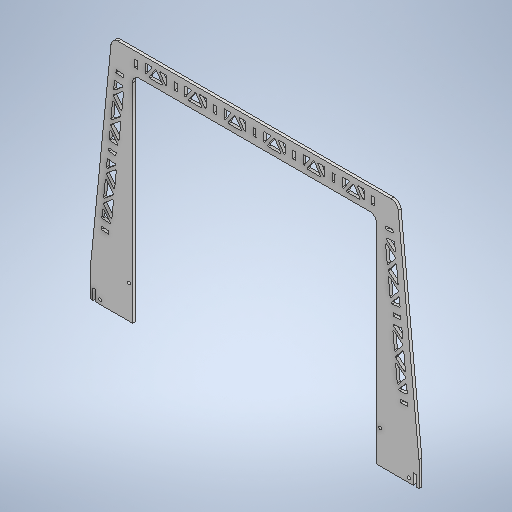
# Autodesk Inventor part: GateBrigeSide
Saved by Autodesk Inventor 2025.1 (Build 291241000, 241)
## iProperties
Created: 2025-03-30
Part Number: GateBrigeSide
Material: Všeobecné
Document SubType Name: Modeling
Designer: 42060
Density: 1 g/cm^3
Appearance: Výchozí
Author: 42060
Autodesk Inventor part; units mm, degrees
ref_plane "YZ Plane" through (0, 0, 0) normal (1, 0, 0) x (0, 1, 0)
ref_plane "XZ Plane" through (0, 0, 0) normal (0, 1, 0) x (-1, 0, 0)
ref_plane "XY Plane" through (0, 0, 0) normal (0, 0, 1) x (1, 0, 0)
sketch "Náčrt1" plane through (0, 0, 0) normal (0, 0, 1) x (1, 0, 0)
  line L0 (0, 0) -> (-160, 0)
  line L1 (-170, -10) -> (-170, -300)
  line L2 (-229, -300) -> (-229, -265.3)
  line L3 (-190.0509, 30) -> (0, 30)
  line L4 (0, 30) -> (0, 0)
  line L5 (-203.7, -249) -> (-170, -249)
  line L6 (-170, -249) -> (-170, -299)
  line L7 (-170, -299) -> (-220, -299)
  line L8 (-220, -299) -> (-220, -265.3)
  line L9 (-220, -265.3) -> (-203.7, -249)
  line L10 (-220, -299) -> (-170, -249) construction
  circle A0 centre (-215, -294) radius 2.1
  circle A1 centre (-175, -254) radius 2.1
  arc A2 (-160, 0) -> (-170, -10) centre (-160, -10) ccw
  line L11 (-200, 21.0077) -> (-229, -265.3)
  arc A3 (-190.0509, 30) -> (-200, 21.0077) centre (-190.0509, 20) ccw
  line L12 (-225, -300) -> (-225, -285)
  line L13 (-225, -285) -> (-221, -285)
  line L14 (-221, -285) -> (-221, -300)
  line L15 (-170, -300) -> (-221, -300)
  line L16 (-225, -300) -> (-229, -300)
  line L17 (-2, 10) -> (2, 10)
  line L18 (2, 10) -> (2, 20)
  line L19 (2, 20) -> (-2, 20)
  line L20 (-2, 20) -> (-2, 10)
  line L21 (-57, 20) -> (-57, 10)
  line L22 (-53, 20) -> (-57, 20)
  line L23 (-53, 10) -> (-53, 20)
  line L24 (-57, 10) -> (-53, 10)
  line L25 (-112, 20) -> (-112, 10)
  line L26 (-108, 20) -> (-112, 20)
  line L27 (-108, 10) -> (-108, 20)
  line L28 (-112, 10) -> (-108, 10)
  line L29 (-167, 20) -> (-167, 10)
  line L30 (-163, 20) -> (-167, 20)
  line L31 (-163, 10) -> (-163, 20)
  line L32 (-167, 10) -> (-163, 10)
  line L33 (-192.6355, -5.5165) -> (-182.6864, -6.5242)
  line L34 (-182.6864, -6.5242) -> (-183.0895, -10.5039)
  line L35 (-183.0895, -10.5039) -> (-193.0386, -9.4961)
  line L36 (-193.0386, -9.4961) -> (-192.6355, -5.5165)
  line L37 (-193.1669, -109.9948) -> (-203.116, -108.9871)
  line L38 (-192.7638, -106.0152) -> (-193.1669, -109.9948)
  line L39 (-203.116, -108.9871) -> (-202.7129, -105.0074)
  line L40 (-202.7129, -105.0074) -> (-192.7638, -106.0152)
  line L41 (-203.2443, -209.4857) -> (-213.1934, -208.478)
  line L42 (-202.8412, -205.5061) -> (-203.2443, -209.4857)
  line L43 (-213.1934, -208.478) -> (-212.7903, -204.4984)
  line L44 (-212.7903, -204.4984) -> (-202.8412, -205.5061)
  line L45 (0, 0) -> (160, 0)
  line L46 (170, -10) -> (170, -300)
  line L47 (229, -300) -> (229, -265.3)
  line L48 (190.0509, 30) -> (0, 30)
  line L49 (203.7, -249) -> (170, -249)
  line L50 (170, -249) -> (170, -299)
  line L51 (170, -299) -> (220, -299)
  line L52 (220, -299) -> (220, -265.3)
  line L53 (220, -265.3) -> (203.7, -249)
  line L54 (220, -299) -> (170, -249) construction
  circle A4 centre (215, -294) radius 2.1
  circle A5 centre (175, -254) radius 2.1
  arc A6 (170, -10) -> (160, 0) centre (160, -10) ccw
  line L55 (200, 21.0077) -> (229, -265.3)
  arc A7 (200, 21.0077) -> (190.0509, 30) centre (190.0509, 20) ccw
  line L56 (225, -300) -> (225, -285)
  line L57 (225, -285) -> (221, -285)
  line L58 (221, -285) -> (221, -300)
  line L59 (170, -300) -> (221, -300)
  line L60 (225, -300) -> (229, -300)
  line L61 (2, 10) -> (-2, 10)
  line L62 (-2, 10) -> (-2, 20)
  line L63 (-2, 20) -> (2, 20)
  line L64 (2, 20) -> (2, 10)
  line L65 (57, 20) -> (57, 10)
  line L66 (53, 20) -> (57, 20)
  line L67 (53, 10) -> (53, 20)
  line L68 (57, 10) -> (53, 10)
  line L69 (112, 20) -> (112, 10)
  line L70 (108, 20) -> (112, 20)
  line L71 (108, 10) -> (108, 20)
  line L72 (112, 10) -> (108, 10)
  line L73 (167, 20) -> (167, 10)
  line L74 (163, 20) -> (167, 20)
  line L75 (163, 10) -> (163, 20)
  line L76 (167, 10) -> (163, 10)
  line L77 (192.6355, -5.5165) -> (182.6864, -6.5242)
  line L78 (182.6864, -6.5242) -> (183.0895, -10.5039)
  line L79 (183.0895, -10.5039) -> (193.0386, -9.4961)
  line L80 (193.0386, -9.4961) -> (192.6355, -5.5165)
  line L81 (193.1669, -109.9948) -> (203.116, -108.9871)
  line L82 (192.7638, -106.0152) -> (193.1669, -109.9948)
  line L83 (203.116, -108.9871) -> (202.7129, -105.0074)
  line L84 (202.7129, -105.0074) -> (192.7638, -106.0152)
  line L85 (203.2443, -209.4857) -> (213.1934, -208.478)
  line L86 (202.8412, -205.5061) -> (203.2443, -209.4857)
  line L87 (213.1934, -208.478) -> (212.7903, -204.4984)
  line L88 (212.7903, -204.4984) -> (202.8412, -205.5061)
  line L89 (-36.6095, 9.0611) -> (-28.3278, 21.2788)
  line L90 (-26.6722, 21.2788) -> (-18.3905, 9.0611)
  line L91 (-19.2183, 7.5) -> (-35.7817, 7.5)
  line L92 (-21.6095, 20.9389) -> (-14.3278, 10.1964)
  line L93 (-12.5, 10.7575) -> (-12.5, 21.5)
  line L94 (-13.5, 22.5) -> (-20.7817, 22.5)
  line L95 (-33.3905, 20.9389) -> (-40.6722, 10.1964)
  line L96 (-42.5, 10.7575) -> (-42.5, 21.5)
  line L97 (-41.5, 22.5) -> (-34.2183, 22.5)
  line L98 (-53, 15) -> (-2, 15) construction
  arc A8 (-41.5, 22.5) -> (-42.5, 21.5) centre (-41.5, 21.5) ccw
  arc A9 (-33.3905, 20.9389) -> (-34.2183, 22.5) centre (-34.2183, 21.5) ccw
  arc A10 (-42.5, 10.7575) -> (-40.6722, 10.1964) centre (-41.5, 10.7575) ccw
  arc A11 (-36.6095, 9.0611) -> (-35.7817, 7.5) centre (-35.7817, 8.5) ccw
  arc A12 (-19.2183, 7.5) -> (-18.3905, 9.0611) centre (-19.2183, 8.5) ccw
  arc A13 (-26.6722, 21.2788) -> (-28.3278, 21.2788) centre (-27.5, 20.7178) ccw
  arc A14 (-20.7817, 22.5) -> (-21.6095, 20.9389) centre (-20.7817, 21.5) ccw
  arc A15 (-12.5, 21.5) -> (-13.5, 22.5) centre (-13.5, 21.5) ccw
  arc A16 (-14.3278, 10.1964) -> (-12.5, 10.7575) centre (-13.5, 10.7575) ccw
  arc A17 (-81.6722, 21.2788) -> (-83.3278, 21.2788) centre (-82.5, 20.7178) ccw
  line L99 (-91.6095, 9.0611) -> (-83.3278, 21.2788)
  line L100 (-68.5, 22.5) -> (-75.7817, 22.5)
  arc A18 (-67.5, 21.5) -> (-68.5, 22.5) centre (-68.5, 21.5) ccw
  line L101 (-81.6722, 21.2788) -> (-73.3905, 9.0611)
  arc A19 (-74.2183, 7.5) -> (-73.3905, 9.0611) centre (-74.2183, 8.5) ccw
  line L102 (-76.6095, 20.9389) -> (-69.3278, 10.1964)
  line L103 (-74.2183, 7.5) -> (-90.7817, 7.5)
  arc A20 (-69.3278, 10.1964) -> (-67.5, 10.7575) centre (-68.5, 10.7575) ccw
  line L104 (-108, 15) -> (-57, 15) construction
  arc A21 (-96.5, 22.5) -> (-97.5, 21.5) centre (-96.5, 21.5) ccw
  arc A22 (-97.5, 10.7575) -> (-95.6722, 10.1964) centre (-96.5, 10.7575) ccw
  arc A23 (-91.6095, 9.0611) -> (-90.7817, 7.5) centre (-90.7817, 8.5) ccw
  arc A24 (-88.3905, 20.9389) -> (-89.2183, 22.5) centre (-89.2183, 21.5) ccw
  line L105 (-67.5, 10.7575) -> (-67.5, 21.5)
  arc A25 (-75.7817, 22.5) -> (-76.6095, 20.9389) centre (-75.7817, 21.5) ccw
  line L106 (-96.5, 22.5) -> (-89.2183, 22.5)
  line L107 (-88.3905, 20.9389) -> (-95.6722, 10.1964)
  line L108 (-97.5, 10.7575) -> (-97.5, 21.5)
  arc A26 (-136.6722, 21.2788) -> (-138.3278, 21.2788) centre (-137.5, 20.7178) ccw
  line L109 (-146.6095, 9.0611) -> (-138.3278, 21.2788)
  line L110 (-123.5, 22.5) -> (-130.7817, 22.5)
  arc A27 (-122.5, 21.5) -> (-123.5, 22.5) centre (-123.5, 21.5) ccw
  line L111 (-136.6722, 21.2788) -> (-128.3905, 9.0611)
  arc A28 (-129.2183, 7.5) -> (-128.3905, 9.0611) centre (-129.2183, 8.5) ccw
  line L112 (-131.6095, 20.9389) -> (-124.3278, 10.1964)
  line L113 (-129.2183, 7.5) -> (-145.7817, 7.5)
  arc A29 (-124.3278, 10.1964) -> (-122.5, 10.7575) centre (-123.5, 10.7575) ccw
  line L114 (-163, 15) -> (-112, 15) construction
  arc A30 (-151.5, 22.5) -> (-152.5, 21.5) centre (-151.5, 21.5) ccw
  arc A31 (-152.5, 10.7575) -> (-150.6722, 10.1964) centre (-151.5, 10.7575) ccw
  arc A32 (-146.6095, 9.0611) -> (-145.7817, 7.5) centre (-145.7817, 8.5) ccw
  arc A33 (-143.3905, 20.9389) -> (-144.2183, 22.5) centre (-144.2183, 21.5) ccw
  line L115 (-122.5, 10.7575) -> (-122.5, 21.5)
  arc A34 (-130.7817, 22.5) -> (-131.6095, 20.9389) centre (-130.7817, 21.5) ccw
  line L116 (-151.5, 22.5) -> (-144.2183, 22.5)
  line L117 (-143.3905, 20.9389) -> (-150.6722, 10.1964)
  line L118 (-152.5, 10.7575) -> (-152.5, 21.5)
  line L119 (-194.0109, -19.4488) -> (-184.1326, -20.4494)
  line L120 (-183.6011, -22.2191) -> (-194.48, -31.0969)
  line L121 (-196.1072, -30.2213) -> (-195.1066, -20.3429)
  line L122 (-182.544, -28.7227) -> (-184.7467, -50.4692)
  line L123 (-186.5164, -51.0007) -> (-196.2883, -39.0261)
  line L124 (-196.1458, -37.6191) -> (-184.1711, -27.8471)
  line L125 (-195.9642, -45.7498) -> (-186.1923, -57.7245)
  line L126 (-186.3348, -59.1315) -> (-198.3095, -68.9034)
  line L127 (-199.9366, -68.0279) -> (-197.7339, -46.2813)
  line L128 (-188.0006, -65.6537) -> (-199.9752, -75.4256)
  line L129 (-200.1177, -76.8326) -> (-190.3458, -88.8073)
  line L130 (-188.5761, -88.2758) -> (-186.3734, -66.5292)
  line L131 (-199.7937, -83.5564) -> (-190.9158, -94.4353)
  line L132 (-191.7914, -96.0625) -> (-201.6698, -95.0619)
  line L133 (-202.5639, -93.9662) -> (-201.5633, -84.0878)
  line L134 (-189.0718, -19.9491) -> (-188.064, -10) construction
  arc A35 (-194.0109, -19.4488) -> (-195.1066, -20.3429) centre (-194.1117, -20.4437) ccw
  arc A36 (-183.6011, -22.2191) -> (-184.1326, -20.4494) centre (-184.2333, -21.4443) ccw
  arc A37 (-196.1072, -30.2213) -> (-194.48, -31.0969) centre (-195.1123, -30.3221) ccw
  arc A38 (-196.1458, -37.6191) -> (-196.2883, -39.0261) centre (-195.5135, -38.3938) ccw
  arc A39 (-186.5164, -51.0007) -> (-184.7467, -50.4692) centre (-185.7416, -50.3685) ccw
  arc A40 (-182.544, -28.7227) -> (-184.1711, -27.8471) centre (-183.5389, -28.6219) ccw
  arc A41 (-195.9642, -45.7498) -> (-197.7339, -46.2813) centre (-196.739, -46.3821) ccw
  arc A42 (-186.3348, -59.1315) -> (-186.1923, -57.7245) centre (-186.9671, -58.3567) ccw
  arc A43 (-199.9366, -68.0279) -> (-198.3095, -68.9034) centre (-198.9417, -68.1287) ccw
  arc A44 (-199.9752, -75.4256) -> (-200.1177, -76.8326) centre (-199.343, -76.2004) ccw
  arc A45 (-190.3458, -88.8073) -> (-188.5761, -88.2758) centre (-189.571, -88.175) ccw
  arc A46 (-186.3734, -66.5292) -> (-188.0006, -65.6537) centre (-187.3683, -66.4284) ccw
  arc A47 (-199.7937, -83.5564) -> (-201.5633, -84.0878) centre (-200.5684, -84.1886) ccw
  arc A48 (-202.5639, -93.9662) -> (-201.6698, -95.0619) centre (-201.569, -94.067) ccw
  arc A49 (-191.7914, -96.0625) -> (-190.9158, -94.4353) centre (-191.6906, -95.0676) ccw
  arc A50 (-212.6413, -193.4572) -> (-211.7472, -194.5528) centre (-211.6464, -193.5579) ccw
  line L135 (-201.8688, -195.5534) -> (-211.7472, -194.5528)
  arc A51 (-201.8688, -195.5534) -> (-200.9932, -193.9263) centre (-201.768, -194.5585) ccw
  arc A52 (-200.4232, -188.2982) -> (-198.6535, -187.7667) centre (-199.6484, -187.666) ccw
  line L136 (-209.871, -183.0473) -> (-200.9932, -193.9263)
  line L137 (-212.6413, -193.4572) -> (-211.6407, -183.5788)
  arc A53 (-209.871, -183.0473) -> (-211.6407, -183.5788) centre (-210.6458, -183.6796) ccw
  line L138 (-198.078, -165.1446) -> (-210.0526, -174.9165)
  line L139 (-210.1951, -176.3236) -> (-200.4232, -188.2982)
  line L140 (-198.6535, -187.7667) -> (-196.4508, -166.0201)
  arc A54 (-210.0526, -174.9165) -> (-210.1951, -176.3236) centre (-209.4204, -175.6913) ccw
  arc A55 (-210.014, -167.5188) -> (-208.3869, -168.3944) centre (-209.0191, -167.6196) ccw
  arc A56 (-196.4508, -166.0201) -> (-198.078, -165.1446) centre (-197.4457, -165.9194) ccw
  line L141 (-206.0416, -145.2407) -> (-196.2697, -157.2154)
  arc A57 (-196.4122, -158.6224) -> (-196.2697, -157.2154) centre (-197.0445, -157.8476) ccw
  line L142 (-210.014, -167.5188) -> (-207.8113, -145.7722)
  line L143 (-196.4122, -158.6224) -> (-208.3869, -168.3944)
  arc A58 (-196.5938, -150.4917) -> (-194.8241, -149.9602) centre (-195.819, -149.8594) ccw
  arc A59 (-206.0416, -145.2407) -> (-207.8113, -145.7722) centre (-206.8164, -145.873) ccw
  line L144 (-196.5938, -150.4917) -> (-206.3657, -138.517)
  arc A60 (-206.2232, -137.11) -> (-206.3657, -138.517) centre (-205.5909, -137.8848) ccw
  arc A61 (-206.1846, -129.7123) -> (-204.5574, -130.5878) centre (-205.1897, -129.813) ccw
  line L145 (-192.6214, -128.2136) -> (-194.8241, -149.9602)
  line L146 (-206.2232, -137.11) -> (-194.2485, -127.338)
  arc A62 (-192.6214, -128.2136) -> (-194.2485, -127.338) centre (-193.6163, -128.1128) ccw
  arc A63 (-193.6785, -121.71) -> (-194.21, -119.9403) centre (-194.3107, -120.9352) ccw
  line L147 (-199.1491, -119.44) -> (-198.1414, -109.4909) construction
  line L148 (-204.0883, -118.9397) -> (-194.21, -119.9403)
  arc A64 (-204.0883, -118.9397) -> (-205.184, -119.8339) centre (-204.1891, -119.9346) ccw
  line L149 (-193.6785, -121.71) -> (-204.5574, -130.5878)
  line L150 (-206.1846, -129.7123) -> (-205.184, -119.8339)
  line L151 (36.6095, 9.0611) -> (28.3278, 21.2788)
  line L152 (26.6722, 21.2788) -> (18.3905, 9.0611)
  line L153 (19.2183, 7.5) -> (35.7817, 7.5)
  line L154 (21.6095, 20.9389) -> (14.3278, 10.1964)
  line L155 (12.5, 10.7575) -> (12.5, 21.5)
  line L156 (13.5, 22.5) -> (20.7817, 22.5)
  line L157 (33.3905, 20.9389) -> (40.6722, 10.1964)
  line L158 (42.5, 10.7575) -> (42.5, 21.5)
  line L159 (41.5, 22.5) -> (34.2183, 22.5)
  line L160 (53, 15) -> (2, 15) construction
  arc A65 (42.5, 21.5) -> (41.5, 22.5) centre (41.5, 21.5) ccw
  arc A66 (34.2183, 22.5) -> (33.3905, 20.9389) centre (34.2183, 21.5) ccw
  arc A67 (40.6722, 10.1964) -> (42.5, 10.7575) centre (41.5, 10.7575) ccw
  arc A68 (35.7817, 7.5) -> (36.6095, 9.0611) centre (35.7817, 8.5) ccw
  arc A69 (18.3905, 9.0611) -> (19.2183, 7.5) centre (19.2183, 8.5) ccw
  arc A70 (28.3278, 21.2788) -> (26.6722, 21.2788) centre (27.5, 20.7178) ccw
  arc A71 (21.6095, 20.9389) -> (20.7817, 22.5) centre (20.7817, 21.5) ccw
  arc A72 (13.5, 22.5) -> (12.5, 21.5) centre (13.5, 21.5) ccw
  arc A73 (12.5, 10.7575) -> (14.3278, 10.1964) centre (13.5, 10.7575) ccw
  line L161 (67.5, 10.7575) -> (67.5, 21.5)
  line L162 (96.5, 22.5) -> (89.2183, 22.5)
  arc A74 (97.5, 21.5) -> (96.5, 22.5) centre (96.5, 21.5) ccw
  line L163 (97.5, 10.7575) -> (97.5, 21.5)
  arc A75 (95.6722, 10.1964) -> (97.5, 10.7575) centre (96.5, 10.7575) ccw
  arc A76 (67.5, 10.7575) -> (69.3278, 10.1964) centre (68.5, 10.7575) ccw
  arc A77 (68.5, 22.5) -> (67.5, 21.5) centre (68.5, 21.5) ccw
  arc A78 (89.2183, 22.5) -> (88.3905, 20.9389) centre (89.2183, 21.5) ccw
  arc A79 (83.3278, 21.2788) -> (81.6722, 21.2788) centre (82.5, 20.7178) ccw
  line L164 (88.3905, 20.9389) -> (95.6722, 10.1964)
  line L165 (91.6095, 9.0611) -> (83.3278, 21.2788)
  arc A80 (76.6095, 20.9389) -> (75.7817, 22.5) centre (75.7817, 21.5) ccw
  arc A81 (90.7817, 7.5) -> (91.6095, 9.0611) centre (90.7817, 8.5) ccw
  line L166 (108, 15) -> (57, 15) construction
  line L167 (68.5, 22.5) -> (75.7817, 22.5)
  line L168 (76.6095, 20.9389) -> (69.3278, 10.1964)
  line L169 (81.6722, 21.2788) -> (73.3905, 9.0611)
  arc A82 (73.3905, 9.0611) -> (74.2183, 7.5) centre (74.2183, 8.5) ccw
  line L170 (74.2183, 7.5) -> (90.7817, 7.5)
  line L171 (122.5, 10.7575) -> (122.5, 21.5)
  line L172 (151.5, 22.5) -> (144.2183, 22.5)
  arc A83 (152.5, 21.5) -> (151.5, 22.5) centre (151.5, 21.5) ccw
  line L173 (152.5, 10.7575) -> (152.5, 21.5)
  arc A84 (150.6722, 10.1964) -> (152.5, 10.7575) centre (151.5, 10.7575) ccw
  arc A85 (122.5, 10.7575) -> (124.3278, 10.1964) centre (123.5, 10.7575) ccw
  arc A86 (123.5, 22.5) -> (122.5, 21.5) centre (123.5, 21.5) ccw
  arc A87 (144.2183, 22.5) -> (143.3905, 20.9389) centre (144.2183, 21.5) ccw
  arc A88 (138.3278, 21.2788) -> (136.6722, 21.2788) centre (137.5, 20.7178) ccw
  line L174 (143.3905, 20.9389) -> (150.6722, 10.1964)
  line L175 (146.6095, 9.0611) -> (138.3278, 21.2788)
  arc A89 (131.6095, 20.9389) -> (130.7817, 22.5) centre (130.7817, 21.5) ccw
  arc A90 (145.7817, 7.5) -> (146.6095, 9.0611) centre (145.7817, 8.5) ccw
  line L176 (163, 15) -> (112, 15) construction
  line L177 (123.5, 22.5) -> (130.7817, 22.5)
  line L178 (131.6095, 20.9389) -> (124.3278, 10.1964)
  line L179 (136.6722, 21.2788) -> (128.3905, 9.0611)
  arc A91 (128.3905, 9.0611) -> (129.2183, 7.5) centre (129.2183, 8.5) ccw
  line L180 (129.2183, 7.5) -> (145.7817, 7.5)
  line L181 (194.0109, -19.4488) -> (184.1326, -20.4494)
  line L182 (183.6011, -22.2191) -> (194.48, -31.0969)
  line L183 (196.1072, -30.2213) -> (195.1066, -20.3429)
  line L184 (182.544, -28.7227) -> (184.7467, -50.4692)
  line L185 (186.5164, -51.0007) -> (196.2883, -39.0261)
  line L186 (196.1458, -37.6191) -> (184.1711, -27.8471)
  line L187 (195.9642, -45.7498) -> (186.1923, -57.7245)
  line L188 (186.3348, -59.1315) -> (198.3095, -68.9034)
  line L189 (199.9366, -68.0279) -> (197.7339, -46.2813)
  line L190 (188.0006, -65.6537) -> (199.9752, -75.4256)
  line L191 (200.1177, -76.8326) -> (190.3458, -88.8073)
  line L192 (188.5761, -88.2758) -> (186.3734, -66.5292)
  line L193 (199.7937, -83.5564) -> (190.9158, -94.4353)
  line L194 (191.7914, -96.0625) -> (201.6698, -95.0619)
  line L195 (202.5639, -93.9662) -> (201.5633, -84.0878)
  line L196 (189.0718, -19.9491) -> (188.064, -10) construction
  arc A92 (195.1066, -20.3429) -> (194.0109, -19.4488) centre (194.1117, -20.4437) ccw
  arc A93 (184.1326, -20.4494) -> (183.6011, -22.2191) centre (184.2333, -21.4443) ccw
  arc A94 (194.48, -31.0969) -> (196.1072, -30.2213) centre (195.1123, -30.3221) ccw
  arc A95 (196.2883, -39.0261) -> (196.1458, -37.6191) centre (195.5135, -38.3938) ccw
  arc A96 (184.7467, -50.4692) -> (186.5164, -51.0007) centre (185.7416, -50.3685) ccw
  arc A97 (184.1711, -27.8471) -> (182.544, -28.7227) centre (183.5389, -28.6219) ccw
  arc A98 (197.7339, -46.2813) -> (195.9642, -45.7498) centre (196.739, -46.3821) ccw
  arc A99 (186.1923, -57.7245) -> (186.3348, -59.1315) centre (186.9671, -58.3567) ccw
  arc A100 (198.3095, -68.9034) -> (199.9366, -68.0279) centre (198.9417, -68.1287) ccw
  arc A101 (200.1177, -76.8326) -> (199.9752, -75.4256) centre (199.343, -76.2004) ccw
  arc A102 (188.5761, -88.2758) -> (190.3458, -88.8073) centre (189.571, -88.175) ccw
  arc A103 (188.0006, -65.6537) -> (186.3734, -66.5292) centre (187.3683, -66.4284) ccw
  arc A104 (201.5633, -84.0878) -> (199.7937, -83.5564) centre (200.5684, -84.1886) ccw
  arc A105 (201.6698, -95.0619) -> (202.5639, -93.9662) centre (201.569, -94.067) ccw
  arc A106 (190.9158, -94.4353) -> (191.7914, -96.0625) centre (191.6906, -95.0676) ccw
  arc A107 (194.21, -119.9403) -> (193.6785, -121.71) centre (194.3107, -120.9352) ccw
  arc A108 (194.2485, -127.338) -> (192.6214, -128.2136) centre (193.6163, -128.1128) ccw
  line L197 (204.0883, -118.9397) -> (194.21, -119.9403)
  line L198 (193.6785, -121.71) -> (204.5574, -130.5878)
  line L199 (206.1846, -129.7123) -> (205.184, -119.8339)
  line L200 (206.2232, -137.11) -> (194.2485, -127.338)
  arc A109 (205.184, -119.8339) -> (204.0883, -118.9397) centre (204.1891, -119.9346) ccw
  arc A110 (204.5574, -130.5878) -> (206.1846, -129.7123) centre (205.1897, -129.813) ccw
  line L201 (192.6214, -128.2136) -> (194.8241, -149.9602)
  arc A111 (207.8113, -145.7722) -> (206.0416, -145.2407) centre (206.8164, -145.873) ccw
  line L202 (196.5938, -150.4917) -> (206.3657, -138.517)
  arc A112 (206.3657, -138.517) -> (206.2232, -137.11) centre (205.5909, -137.8848) ccw
  arc A113 (194.8241, -149.9602) -> (196.5938, -150.4917) centre (195.819, -149.8594) ccw
  line L203 (206.0416, -145.2407) -> (196.2697, -157.2154)
  arc A114 (196.2697, -157.2154) -> (196.4122, -158.6224) centre (197.0445, -157.8476) ccw
  arc A115 (198.078, -165.1446) -> (196.4508, -166.0201) centre (197.4457, -165.9194) ccw
  line L204 (196.4122, -158.6224) -> (208.3869, -168.3944)
  arc A116 (208.3869, -168.3944) -> (210.014, -167.5188) centre (209.0191, -167.6196) ccw
  line L205 (210.014, -167.5188) -> (207.8113, -145.7722)
  arc A117 (200.9932, -193.9263) -> (201.8688, -195.5534) centre (201.768, -194.5585) ccw
  arc A118 (211.7472, -194.5528) -> (212.6413, -193.4572) centre (211.6464, -193.5579) ccw
  arc A119 (198.6535, -187.7667) -> (200.4232, -188.2982) centre (199.6484, -187.666) ccw
  line L206 (212.6413, -193.4572) -> (211.6407, -183.5788)
  line L207 (209.871, -183.0473) -> (200.9932, -193.9263)
  arc A120 (211.6407, -183.5788) -> (209.871, -183.0473) centre (210.6458, -183.6796) ccw
  line L208 (210.1951, -176.3236) -> (200.4232, -188.2982)
  arc A121 (210.1951, -176.3236) -> (210.0526, -174.9165) centre (209.4204, -175.6913) ccw
  line L209 (198.6535, -187.7667) -> (196.4508, -166.0201)
  line L210 (198.078, -165.1446) -> (210.0526, -174.9165)
  line L211 (201.8688, -195.5534) -> (211.7472, -194.5528)
  line L212 (-42.5, 10.7575) -> (-42.5, 7.5) construction
  line L213 (-42.5, 7.5) -> (-40.6722, 10.1964) construction
  line L214 (-27.5, 22.5) -> (-27.5, 7.5) construction
  point P0 (2, 15)
  point P1 (0, 15)
  point P2 (0, 10)
  point P3 (-55, 10)
  point P4 (-110, 10)
  point P5 (-165, 10)
  point P6 (55, 10)
  point P7 (108, 15)
  point P8 (110, 10)
  point P9 (163, 15)
  point P10 (165, 10)
  point P11 (-12.5, 7.5)
  point P12 (-32.3323, 22.5)
  point P13 (-42.5, 22.5)
  point P14 (-27.5, 15)
  point P15 (-12.5, 16.1288)
  point P16 (-2, 15)
  point P17 (-82.5, 22.5)
  point P18 (-82.5, 15)
  point P19 (-82.5, 7.5)
  point P20 (-87.3323, 22.5)
  point P21 (-97.5, 22.5)
  point P22 (-67.5, 7.5)
  point P23 (-67.5, 16.1288)
  point P24 (-137.5, 22.5)
  point P25 (-137.5, 15)
  point P26 (-137.5, 7.5)
  point P27 (-142.3323, 22.5)
  point P28 (-152.5, 22.5)
  point P29 (-122.5, 7.5)
  point P30 (-122.5, 16.1288)
  point P31 (-195.0059, -19.348)
  point P32 (-181.7306, -20.6927)
  point P33 (-196.3505, -32.6233)
  point P34 (-182.3007, -26.3207)
  point P35 (-184.99, -52.8712)
  point P36 (-196.9206, -38.2513)
  point P37 (-197.4906, -43.8794)
  point P38 (-185.56, -58.4992)
  point P39 (-200.1799, -70.4298)
  point P40 (-186.1301, -64.1273)
  point P41 (-200.75, -76.0579)
  point P42 (-188.8194, -90.6777)
  point P43 (-201.32, -81.6859)
  point P44 (-189.3895, -96.3058)
  point P45 (-202.6647, -94.9611)
  point P46 (-212.7421, -194.4521)
  point P47 (-199.4669, -195.7967)
  point P48 (-198.8968, -190.1687)
  point P49 (-211.3974, -181.1769)
  point P50 (-210.8274, -175.5488)
  point P51 (-210.2573, -169.9207)
  point P52 (-196.2075, -163.6182)
  point P53 (-195.6374, -157.9902)
  point P54 (-195.0674, -152.3621)
  point P55 (-207.568, -143.3703)
  point P56 (-206.998, -137.7422)
  point P57 (-206.4279, -132.1142)
  point P58 (-192.3781, -125.8117)
  point P59 (-191.808, -120.1836)
  point P60 (-205.0833, -118.839)
  point P61 (27.5, 22.5)
  point P62 (12.5, 7.5)
  point P63 (32.3323, 22.5)
  point P64 (42.5, 22.5)
  point P65 (27.5, 7.5)
  point P66 (27.5, 15)
  point P67 (12.5, 16.1288)
  point P68 (67.5, 7.5)
  point P69 (67.5, 16.1288)
  point P70 (82.5, 22.5)
  point P71 (87.3323, 22.5)
  point P72 (97.5, 22.5)
  point P73 (82.5, 15)
  point P74 (82.5, 7.5)
  point P75 (122.5, 7.5)
  point P76 (122.5, 16.1288)
  point P77 (137.5, 22.5)
  point P78 (142.3323, 22.5)
  point P79 (152.5, 22.5)
  point P80 (137.5, 15)
  point P81 (137.5, 7.5)
  point P82 (195.0059, -19.348)
  point P83 (181.7306, -20.6927)
  point P84 (196.3505, -32.6233)
  point P85 (182.3007, -26.3207)
  point P86 (184.99, -52.8712)
  point P87 (196.9206, -38.2513)
  point P88 (197.4906, -43.8794)
  point P89 (185.56, -58.4992)
  point P90 (200.1799, -70.4298)
  point P91 (186.1301, -64.1273)
  point P92 (200.75, -76.0579)
  point P93 (188.8194, -90.6777)
  point P94 (201.32, -81.6859)
  point P95 (189.3895, -96.3058)
  point P96 (202.6647, -94.9611)
  point P97 (191.808, -120.1836)
  point P98 (192.3781, -125.8117)
  point P99 (199.1491, -119.44)
  point P100 (205.0833, -118.839)
  point P101 (206.4279, -132.1142)
  point P102 (206.998, -137.7422)
  point P103 (195.0674, -152.3621)
  point P104 (207.568, -143.3703)
  point P105 (195.6374, -157.9902)
  point P106 (196.2075, -163.6182)
  point P107 (210.2573, -169.9207)
  point P108 (212.7421, -194.4521)
  point P109 (199.4669, -195.7967)
  point P110 (198.8968, -190.1687)
  point P111 (210.8274, -175.5488)
  point P112 (211.3974, -181.1769)
  point P113 (-27.5, 15)
  dimension "d0" = 50
  dimension "d1" = 50
  dimension "d3" = 33.7
  dimension "d4" = 45
  dimension "d5" = 0
  dimension "d6" = 4.2
  dimension "d7" = 5
  dimension "d8" = 5
  dimension "d10" = 170
  dimension "d12" = 30
  dimension "d14" = 10
  dimension "d16" = 15
  dimension "d17" = 1
  dimension "d18" = 4
  dimension "d19" = 1
  dimension "d20" = 4
  dimension "d21" = 300
  dimension "d22" = 30
  dimension "d25" = 4
  dimension "d26" = 10
  dimension "d29" = 55
  dimension "d34" = 4
  dimension "d35" = 10
  dimension "d36" = 10
  dimension "d39" = 100
  dimension "d46" = 4
  dimension "d47" = 4
  dimension "d50" = 15
  dimension "d51" = 30
  dimension "d52" = 1
  dimension "d55" = 55
  dimension "d60" = 10
  dimension "d61" = 10
  dimension "d63" = 4
  dimension "d64" = 4
  dimension "d65" = 4
  dimension "d66" = 4
  dimension "d67" = 1
  dimension "d70" = 100
  dimension "d77" = 55
  dimension "d84" = 100
  constraints: 430 end point, 236 point on circle, 212 point on line, 152 symmetric about line, 122 centre point, 52 tangent, 24 equal radius, 18 perpendicular, 17 parallel, 10 midpoint, 8 collinear, 8 horizontal, 5 horizontal alignment, 3 vertical, 3 vertical alignment, 2 equal length, 481 other
  measures "d0" distance of L5.end L6.end
  measures "d1" distance of L6.end L7.end
  measures "d3" distance of L5.start L5.end
  measures "d4" angle of L5 L9
  measures "d5" distance between parallel lines of L1 L6
  measures "d6" diameter of A1
  measures "d7" distance from line of L5 A1.centre
  measures "d8" distance from line of L7 A0.centre
  measures "d10" distance between parallel lines of L1 L4
  measures "d12" distance between parallel lines of L0 L3
  measures "d14" radius of A3
  measures "d16" distance between parallel lines of L16 L13
  measures "d17" distance between parallel lines of L7 L15
  measures "d18" distance between parallel lines of L14 L12
  measures "d19" distance between parallel lines of L8 L14
  measures "d20" distance between parallel lines of L12 L2
  measures "d21" distance between parallel lines of L15 L0
  measures "d22" distance from line of L11.start L1
  measures "d25" distance of L18.end L19.end
  measures "d26" distance of L17.end L18.end
  measures "d29" distance of L19.end L21.start
  measures "d34" distance of L35.end L33.start
  measures "d35" distance of L33.start L33.end
  measures "d36" distance between parallel lines of L11 L36
  measures "d39" distance of L34.end L37.start
  measures "d46" distance between parallel lines of L89 L95
  measures "d47" distance between parallel lines of L92 L90
  measures "d50" distance from line of L91 L214.start
  measures "d51" distance between parallel lines of L93 L96
  measures "d52" radius of A8
  measures "d55" distance of L214.start point (-82.5, 22.5)
  measures "d60" distance between parallel lines of L35 L119
  measures "d61" distance between parallel lines of L132 L40
  measures "d63" distance between parallel lines of L124 L120
  measures "d64" distance between parallel lines of L125 L123
  measures "d65" distance between parallel lines of L128 L126
  measures "d66" distance between parallel lines of L129 L131
  measures "d67" radius of A35
  measures "d70" distance of point (-202.665, -94.961) point (-212.742, -194.452)
  measures "d77" distance of point (12.5, 7.5) point (67.5, 7.5)
  measures "d84" distance of point (181.731, -20.693) point (191.808, -120.184)
extrude "Vysunutí1" add sketch "Náčrt1" along normal blind 4 contours L0 A2 L1 L5 L9 L8 L7 L15 L14 L13 L12 L16 L2 L11 A3 L3 L4 L19 L20 L17 | L4 L17 L18 L19 L48 A7 L55 L47 L60 L56 L57 L58 L59 L46 L51 L52 L53 L49 A6 L45 | L1 L7 L8 L9 L5 | L49 L53 L52 L51 L46
equation "\"d25\" = d18"
equation "\"d34\" = d18"
equation "\"d35\" = d26"
equation "\"d36\" = d26"
equation "\"d44\" = d18"
